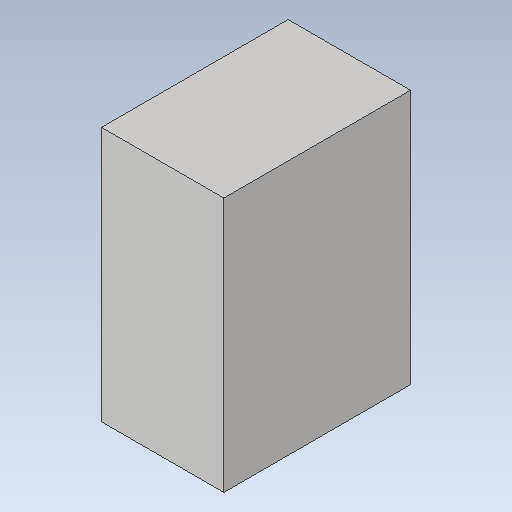
# Autodesk Inventor part: Box
Saved by Autodesk Inventor 2020.1 (Build 241239000, 239)
## iProperties
Created: 2019-05-07
Part Number: Box
Material: Generic
Document SubType Name: Modeling
Designer: Adam Nagy
Density: 1 g/cm^3
Appearance: Default
Author: Adam Nagy
Autodesk Inventor part; units mm, degrees
ref_plane "YZ Plane" through (0, 0, 0) normal (1, 0, 0) x (0, 1, 0)
ref_plane "XZ Plane" through (0, 0, 0) normal (0, 1, 0) x (-1, 0, 0)
ref_plane "XY Plane" through (0, 0, 0) normal (0, 0, 1) x (1, 0, 0)
sketch "Sketch1" plane through (0, 0, 0) normal (0, 1, 0) x (-1, 0, 0)
  line L0 (0, 0) -> (-12.1908, 0)
  line L1 (-12.1908, 0) -> (-12.1908, -18.6015)
  line L2 (-12.1908, -18.6015) -> (0, -18.6015)
  line L3 (0, -18.6015) -> (0, 0)
  constraints: 8 end point, 2 parallel, 1 horizontal, 1 perpendicular
extrude "Extrusion1" add sketch "Sketch1" along normal blind 25.4
body "Solid1"
